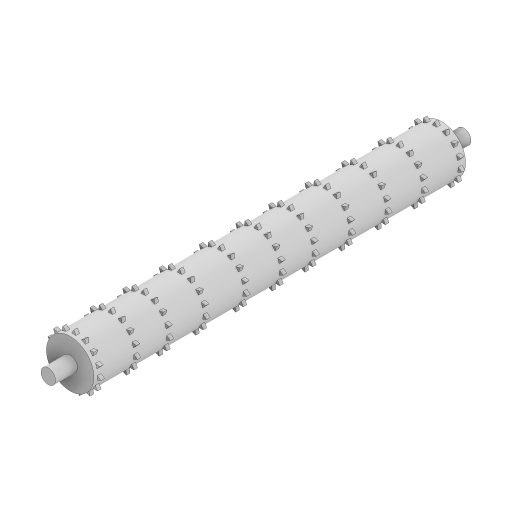
# Autodesk Inventor part: RODILLO
Saved by Autodesk Inventor 2024 (Build 280153000, 153)
## iProperties
Created: 2024-06-28
Part Number: RODILLO
Material: Generic
Document SubType Name: Modeling
Designer: Jhuliams
Density: 1 g/cm^3
Appearance: Default
Author: Jhuliams
Autodesk Inventor part; units mm, degrees
ref_plane "YZ Plane" through (0, 0, 0) normal (1, 0, 0) x (0, 1, 0)
ref_plane "XZ Plane" through (0, 0, 0) normal (0, 1, 0) x (-1, 0, 0)
ref_plane "XY Plane" through (0, 0, 0) normal (0, 0, 1) x (1, 0, 0)
sketch "Sketch1" plane through (0, 0, 0) normal (0, 0, 1) x (1, 0, 0)
  circle A0 centre (0, 0) radius 30
  circle A1 centre (0, 0) radius 32.5
  dimension "d0" = 60
  dimension "d1" = 65
  constraints: 2 centre point, 2 coincident
  measures "d0" diameter of A0
  measures "d1" diameter of A1
extrude "Extrusion1" add sketch "Sketch1" along normal blind 500
ref_plane "Work Plane9" through (0, 0, 50) normal (0, 0, 1) x (1, 0, 0)
ref_plane "Work Plane8" through (0, 0, 100) normal (0, 0, 1) x (1, 0, 0)
sketch "Sketch2" plane through (0, 0, 500) normal (0, 0, 1) x (1, 0, 0)
  line L0 (0, 0) -> (0, 37.5)
  line L1 (0, 37.5) -> (-2.965, 32.3645)
  line L2 (0, 37.5) -> (13.9719, 37.5)
  line L3 (0, 37.5) -> (2.965, 32.3645)
  circle A0 centre (0, 0) radius 32.5
  line L4 (-15.2526, 34.258) -> (-15.8725, 28.3604)
  line L5 (-15.2526, 34.258) -> (-10.4552, 30.7724)
  line L6 (-27.8679, 25.0924) -> (-26.0355, 19.4526)
  line L7 (-27.8679, 25.0924) -> (-22.0675, 23.8595)
  line L8 (-35.6646, 11.5881) -> (-31.6967, 7.1813)
  line L9 (-35.6646, 11.5881) -> (-29.8642, 12.8211)
  line L10 (-37.2946, -3.9198) -> (-31.8772, -6.3318)
  line L11 (-37.2946, -3.9198) -> (-32.4971, -0.4342)
  line L12 (-32.476, -18.75) -> (-26.546, -18.75)
  line L13 (-32.476, -18.75) -> (-29.511, -13.6145)
  line L14 (-22.0419, -30.3381) -> (-16.6246, -27.9262)
  line L15 (-22.0419, -30.3381) -> (-21.4221, -24.4406)
  line L16 (-7.7967, -36.6805) -> (-3.8287, -32.2737)
  line L17 (-7.7967, -36.6805) -> (-9.6292, -31.0408)
  line L18 (7.7967, -36.6805) -> (9.6292, -31.0408)
  line L19 (7.7967, -36.6805) -> (3.8287, -32.2737)
  line L20 (22.0419, -30.3381) -> (21.4221, -24.4406)
  line L21 (22.0419, -30.3381) -> (16.6246, -27.9262)
  line L22 (32.476, -18.75) -> (29.511, -13.6145)
  line L23 (32.476, -18.75) -> (26.546, -18.75)
  line L24 (37.2946, -3.9198) -> (32.4971, -0.4342)
  line L25 (37.2946, -3.9198) -> (31.8772, -6.3318)
  line L26 (35.6646, 11.5881) -> (29.8642, 12.8211)
  line L27 (35.6646, 11.5881) -> (31.6967, 7.1813)
  line L28 (27.8679, 25.0924) -> (22.0675, 23.8595)
  line L29 (27.8679, 25.0924) -> (26.0355, 19.4526)
  line L30 (15.2526, 34.258) -> (10.4552, 30.7724)
  line L31 (15.2526, 34.258) -> (15.8725, 28.3604)
  point P0 (-6.9859, 25.4)
  point P1 (6.9859, 25.4)
  dimension "d15" = 65
  dimension "d13" = 37.5
  dimension "d14" = 120
  dimension "d18" = 360
  constraints: 64 end point, 1 coincident, 1 horizontal, 1 symmetric about line, 1 vertical, 80 other
  measures "d13" distance of L0.start L0.end
  measures "d14" angle of L1 L2
extrude "Extrusion2" add sketch "Sketch2" against normal blind 5 contours A0 L1 L0 | L0 L3 A0 | L30 L31 A0 | A0 L4 L5 | L28 L29 A0 | A0 L6 L7 | L26 L27 A0 | A0 L8 L9 | A0 L10 L11 | L24 L25 A0 | A0 L12 L13 | L22 L23 A0 | A0 L14 L15 | L20 L21 A0 | A0 L16 L17 | L18 L19 A0
mirror "Mirror1" about plane through (0, 0, 450) normal (0, 0, 1) of "Extrusion2"
mirror "Mirror2" about plane through (0, 0, 350) normal (0, 0, 1) of "Extrusion2", "Mirror1"
mirror "Mirror3" about plane through (0, 0, 300) normal (0, 0, 1) of "Extrusion2"
mirror "Mirror4" about plane through (0, 0, 250) normal (0, 0, 1) of "Extrusion2"
sketch "Sketch5" plane through (0, 0, 450) normal (0, 0, 1) x (1, 0, 0)
  line L0 (0, 0) -> (0, 37.5)
  line L1 (0, 37.5) -> (-2.965, 32.3645)
  line L2 (0, 37.5) -> (13.9719, 37.5)
  line L3 (0, 37.5) -> (2.965, 32.3645)
  circle A0 centre (0, 0) radius 32.5
  line L4 (-15.2526, 34.258) -> (-15.8725, 28.3604)
  line L5 (-15.2526, 34.258) -> (-10.4552, 30.7724)
  line L6 (-27.8679, 25.0924) -> (-26.0355, 19.4526)
  line L7 (-27.8679, 25.0924) -> (-22.0675, 23.8595)
  line L8 (-35.6646, 11.5881) -> (-31.6967, 7.1813)
  line L9 (-35.6646, 11.5881) -> (-29.8642, 12.8211)
  line L10 (-37.2946, -3.9198) -> (-31.8772, -6.3318)
  line L11 (-37.2946, -3.9198) -> (-32.4971, -0.4342)
  line L12 (-32.476, -18.75) -> (-26.546, -18.75)
  line L13 (-32.476, -18.75) -> (-29.511, -13.6145)
  line L14 (-22.0419, -30.3381) -> (-16.6246, -27.9262)
  line L15 (-22.0419, -30.3381) -> (-21.4221, -24.4406)
  line L16 (-7.7967, -36.6805) -> (-3.8287, -32.2737)
  line L17 (-7.7967, -36.6805) -> (-9.6292, -31.0408)
  line L18 (7.7967, -36.6805) -> (9.6292, -31.0408)
  line L19 (7.7967, -36.6805) -> (3.8287, -32.2737)
  line L20 (22.0419, -30.3381) -> (21.4221, -24.4406)
  line L21 (22.0419, -30.3381) -> (16.6246, -27.9262)
  line L22 (32.476, -18.75) -> (29.511, -13.6145)
  line L23 (32.476, -18.75) -> (26.546, -18.75)
  line L24 (37.2946, -3.9198) -> (32.4971, -0.4342)
  line L25 (37.2946, -3.9198) -> (31.8772, -6.3318)
  line L26 (35.6646, 11.5881) -> (29.8642, 12.8211)
  line L27 (35.6646, 11.5881) -> (31.6967, 7.1813)
  line L28 (27.8679, 25.0924) -> (22.0675, 23.8595)
  line L29 (27.8679, 25.0924) -> (26.0355, 19.4526)
  line L30 (15.2526, 34.258) -> (10.4552, 30.7724)
  line L31 (15.2526, 34.258) -> (15.8725, 28.3604)
  point P0 (0, 0)
  point P1 (-6.9859, 25.4)
  point P2 (6.9859, 25.4)
  dimension "d26" = 65
  dimension "d24" = 37.5
  dimension "d25" = 120
  dimension "d27" = 360
  constraints: 64 end point, 1 coincident, 1 horizontal, 1 symmetric about line, 1 vertical, 80 other
  measures "d24" distance of L0.start L0.end
  measures "d25" angle of L1 L2
extrude "Extrusion3" add sketch "Sketch5" against normal blind 5 contours A0 L1 L0 | L0 L3 A0 | L30 L31 A0 | A0 L4 L5 | L28 L29 A0 | A0 L6 L7 | L26 L27 A0 | A0 L8 L9 | A0 L10 L11 | L24 L25 A0 | A0 L12 L13 | L22 L23 A0 | A0 L14 L15 | L20 L21 A0 | A0 L16 L17 | L18 L19 A0
mirror "Mirror5" about plane through (0, 0, 400) normal (0, 0, 1) of "Extrusion3"
mirror "Mirror6" about plane through (0, 0, 300) normal (0, 0, 1) of "Extrusion3", "Mirror5"
mirror "Mirror7" about plane through (0, 0, 250) normal (0, 0, 1) of "Extrusion3"
sketch "Sketch6" plane through (0, 0, 500) normal (0, 0, 1) x (1, 0, 0)
  circle A0 centre (0, 0) radius 32.5
  dimension "d30" = 65
  constraints: 1 centre point, 1 coincident
  measures "d30" diameter of A0
extrude "Extrusion4" add sketch "Sketch6" along normal blind 5
sketch "Sketch7" plane through (0, 0, 505) normal (0, 0, 1) x (1, 0, 0)
  circle A0 centre (0, 0) radius 10
  dimension "d33" = 20
  constraints: 1 centre point, 1 coincident
  measures "d33" diameter of A0
extrude "Extrusion5" add sketch "Sketch7" along normal blind 30
mirror "Mirror8" about plane through (0, 0, 250) normal (0, 0, 1) of "Extrusion4", "Extrusion5"
ref_plane "Work Plane1" through (0, 0, 450) normal (0, 0, 1) x (1, 0, 0)
ref_plane "Work Plane2" through (0, 0, 400) normal (0, 0, 1) x (1, 0, 0)
ref_plane "Work Plane3" through (0, 0, 350) normal (0, 0, 1) x (1, 0, 0)
ref_plane "Work Plane4" through (0, 0, 300) normal (0, 0, 1) x (1, 0, 0)
ref_plane "Work Plane5" through (0, 0, 250) normal (0, 0, 1) x (1, 0, 0)
ref_plane "Work Plane6" through (0, 0, 200) normal (0, 0, 1) x (1, 0, 0)
ref_plane "Work Plane7" through (0, 0, 150) normal (0, 0, 1) x (1, 0, 0)
body "Solid1"
